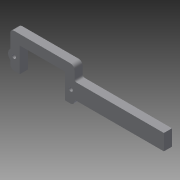
# Autodesk Inventor part: Fork
Saved by Autodesk Inventor 2014 SP1 (Build 180222100, 222)
## iProperties
Created: 2017-01-16
Part Number: Fork
Material: Generic
Document SubType Name: Modeling
Designer: danielsikar
Density: 1 g/cm^3
Appearance: Default
Author: danielsikar
Autodesk Inventor part; units mm, degrees
ref_plane "YZ Plane" through (0, 0, 0) normal (1, 0, 0) x (0, 1, 0)
ref_plane "XZ Plane" through (0, 0, 0) normal (0, 1, 0) x (-1, 0, 0)
sketch "Sketch1" plane through (0, 0, 0) normal (0, 0, 1) x (1, 0, 0)
  line L0 (0, 0) -> (22.8, 0) projected
  line L1 (22.8, 0) -> (22.8, 15.6) projected
  line L2 (22.8, 15.6) -> (27.6, 15.6) projected
  line L3 (27.6, 18) -> (27.6, 15.6) projected
  line L4 (22.8, 18) -> (27.6, 18) projected
  line L5 (22.8, 18) -> (22.8, 22.1) projected
  line L6 (6.25, 22.1) -> (22.8, 22.1) projected
  line L7 (0, 22.1) -> (6.25, 22.1) projected
  line L8 (0, 18) -> (0, 22.1) projected
  line L9 (0, 18) -> (-4.8, 18) projected
  line L10 (-4.8, 18) -> (-4.8, 15.6) projected
  line L11 (0, 15.6) -> (-4.8, 15.6) projected
  line L12 (0, 0) -> (0, 15.6) projected
  line L13 (27.6, 18) -> (22.8, 18)
  line L14 (22.8, 18) -> (22.8, 22.1)
  line L15 (22.8, 22.1) -> (27.6, 22.1)
  line L16 (27.6, 22.1) -> (27.6, 18)
  line L17 (0, 22.1) -> (-4.8, 22.1)
  line L18 (-4.8, 22.1) -> (-4.8, 18)
  line L19 (-4.8, 18) -> (0, 18)
  line L20 (0, 18) -> (0, 22.1)
  constraints: 16 end point, 4 parallel, 2 horizontal, 2 perpendicular
ref_plane "Work Plane1" through (-4.8, 0, -12.5) normal (0, 0, -1) x (0, 1, 0)
extrude "Extrusion1" add sketch "Sketch1" against normal up to surface (12.5 mm away) contours L18 L17 L8 L9 | L4 L5 L15 L16
sketch "Sketch6" plane through (0, 0, 0) normal (0, 0, 1) x (1, 0, 0)
  line L0 (27.6, 22.1) -> (-4.8, 22.1)
  line L1 (-4.8, 22.1) -> (-4.8, 18)
  line L2 (-4.8, 18) -> (27.6, 18)
  line L3 (27.6, 18) -> (27.6, 22.1)
  point P0 (0, 0)
  dimension "d8" = 32.4
  dimension "d9" = 4.1
  constraints: 8 end point, 2 parallel, 1 horizontal, 1 perpendicular
  measures "d8" distance of L2.end L1.end
  measures "d9" distance of L1.end L0.end
extrude "Extrusion5" add sketch "Sketch6" along normal blind 5
sketch "Sketch7" plane through (22.8, 18, -12.5) normal (0, -1, 0) x (1, 0, 0)
  arc A0 (3.7, 6.85) -> (3.7, 5.65) centre (2.9, 6.25) ccw projected
  circle A1 centre (2.9, 6.25) radius 1
  constraints: 1 centre point, 1 coincident, 1 concentric
extrude "Extrusion6" cut sketch "Sketch7" against normal blind 4.1
sketch "Sketch8" plane through (22.8, 18, -12.5) normal (0, -1, 0) x (1, 0, 0)
  arc A0 (-26.5, 5.65) -> (-26.5, 6.85) centre (-25.7, 6.25) ccw projected
  circle A1 centre (-25.7, 6.25) radius 1
  constraints: 1 centre point, 1 coincident, 1 concentric
extrude "Extrusion7" cut sketch "Sketch8" against normal blind 4.1
sketch "Sketch9" plane through (27.6, 18, -12.5) normal (1, 0, 0) x (0, 0, -1)
  line L0 (0, 0) -> (0, 4.1) projected
  line L1 (0, 4.1) -> (-17.5, 4.1) projected
  line L2 (-17.5, 0) -> (0, 0) projected
  line L3 (-10.65, 4.1) -> (-2.65, 4.1)
  line L4 (-2.65, 4.1) -> (-2.65, 0)
  line L5 (-2.65, 0) -> (-10.65, 0)
  line L6 (-10.65, 0) -> (-10.65, 4.1)
  point P0 (-12.5, -18)
  dimension "d16" = 8
  dimension "d17" = 2.65
  constraints: 8 end point, 2 parallel, 2 point on line, 1 horizontal, 1 perpendicular
  measures "d16" distance of L4.end L5.end
  measures "d17" distance between parallel lines of L0 L4
extrude "Extrusion8" add sketch "Sketch9" along normal blind 45 contours L2 L6 L1 L4
fillet "Fillet1" radius 2 4 edges at (27.6, 20.05, 5) (-4.8, 20.05, 5) (-4.8, 20.05, -12.5) (27.6, 20.05, -12.5)
fillet "Fillet2" radius 1 2 edges at (27.6, 20.05, -1.85) (27.6, 20.05, -9.85)
sketch "Sketch14" plane through (0, 22.1, 0) normal (0, 1, 0) x (1, 0, 0)
  circle A0 centre (-2.9, 6.25) radius 1 projected
  arc A1 (-4.8, 8.5716) -> (-4.8, 3.9284) centre (-2.9, 6.25) ccw
  line L0 (-4.8, 8.5716) -> (-4.8, 3.9284)
  dimension "d30" = 6
  constraints: 2 end point, 2 point on circle, 1 centre point, 1 coincident
  measures "d30" diameter of A1
extrude "Extrusion13" add sketch "Sketch14" against normal up to surface (4.1 mm away) contours L0 A1
body "Solid1"
